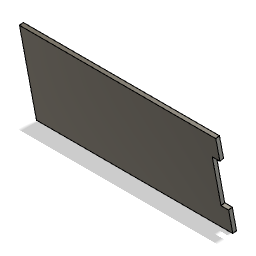
Roof Top 36 x 72 mm screen PCB v7 (Autodesk Fusion 360 design; units mm, degrees)
Autodesk Fusion 360 part; units mm, degrees
sketch "Sketch1" plane through (0, -7.0615, 37.6569) normal (0, 0.18431, -0.982868) x (-1, 0, 0)
  line L0 (2.114, 30.6323) -> (-81.886, 30.6323)
  line L1 (-81.886, 30.6323) -> (-81.886, 20.8412)
  line L2 (-81.886, 20.8412) -> (-78.636, 20.8412)
  line L3 (-78.636, 20.8412) -> (-78.636, 28.8412)
  line L4 (-78.636, 28.8412) -> (-6.636, 28.8412)
  line L5 (-6.636, 28.8412) -> (-6.636, -7.4588)
  line L6 (-6.636, -7.4588) -> (-78.636, -7.4588)
  line L7 (-78.636, -7.4588) -> (-78.636, 0.5412)
  line L8 (-78.636, 0.5412) -> (-81.886, 0.5412)
  line L9 (-81.886, 0.5412) -> (-81.886, -10.9695)
  ellipse E0 centre (-79.886, -13.2445) end of major axis (-79.886, -16.2968) minor radius 3 (-76.9458, -12.6383) -> (-81.886, -10.9695) ccw
  line L10 (-76.9458, -12.6383) -> (-76.9458, -9.6383)
  line L11 (-76.9458, -9.6383) -> (-2.8262, -9.6383)
  line L12 (-2.8262, -9.6383) -> (-2.8262, -12.6383)
  ellipse E1 centre (0.114, -13.2445) end of major axis (0.114, -16.2968) minor radius 3 (2.114, -10.9695) -> (-2.8262, -12.6383) ccw
  line L13 (2.114, -10.9695) -> (2.114, 30.6323)
  line L14 (-78.636, 0.5412) -> (-78.636, -7.4588)
  line L15 (-78.636, -7.4588) -> (-6.636, -7.4588)
  line L16 (-6.636, -7.4588) -> (-6.636, 28.8412)
  line L17 (-6.636, 28.8412) -> (-78.636, 28.8412)
  line L18 (-78.636, 28.8412) -> (-78.636, 20.8412)
  line L19 (-78.636, 20.8412) -> (-81.886, 20.8412)
  line L20 (-81.886, 20.8412) -> (-81.886, 0.5412)
  line L21 (-81.886, 0.5412) -> (-78.636, 0.5412)
  line L22 (-70.636, 26.6912) -> (-9.136, 26.6912)
  line L23 (-9.136, 26.6912) -> (-9.136, -5.3088)
  line L24 (-9.136, -5.3088) -> (-70.636, -5.3088)
  line L25 (-70.636, -5.3088) -> (-70.636, 26.6912)
  line L26 (-76.9458, -9.6383) -> (-81.886, -9.6383)
  line L27 (-2.8262, -9.6383) -> (2.114, -9.6383)
  line L28 (-78.636, 20.8412) -> (-78.636, 0.5412)
  constraint coincident L10.end L11.start
  constraint coincident L9 L26.end
  constraint perpendicular L9 L26
  constraint coincident L11.end L12.start
  constraint coincident L13 L27.end
  constraint perpendicular L13 L27
  constraint coincident L2.end L3.start
  constraint coincident L7.end L8.start
extrude "Extrude1" add sketch "Sketch1" along normal blind 1.6 contours L0 L1 L2 L3 L4 L5 L6 L7 L8 L9 L11 L13 L14 L15 L16 L17 L18 L19 L21 L26 L27 | L3 L4 L5 L6 L7 L14 L15 L16 L17 L18 L28 | L22 L23 L24 L25
extrude "Extrude2" cut 1 faces at (53.886, 23.2426, 42.2544) along direction (0, -0.982868, -0.18431) blind 0.05
extrude "Extrude3" cut 1 faces at (53.886, -16.4364, 35.3563) along direction (0, 0.982868, 0.18431) blind 0.05
extrude "Extrude4" cut 1 faces at (53.886, 23.1934, 42.2452) along direction (0, -0.982868, -0.18431) blind 0.05
extrude "Extrude5" cut 1 faces at (53.886, -16.3873, 35.3655) along direction (0, 0.982868, 0.18431) blind 0.05
extrude "Extrude6" cut 1 faces at (53.886, -16.3382, 35.3747) along direction (0, 0.982868, 0.18431) blind 0.5
extrude "Extrude7" cut 1 faces at (53.886, 23.1443, 42.236) along direction (0, -0.982868, -0.18431) blind 0.5
extrude "Extrude8" add 1 faces at (53.886, 22.6528, 42.1438) along direction (0, 0.982868, 0.18431) blind 0.2
extrude "Extrude9" add 1 faces at (53.886, -15.8467, 35.4669) along direction (0, -0.982868, -0.18431) blind 0.2
